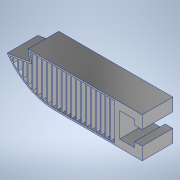
# Autodesk Inventor part: Finray_9_Kerbe_10deg
Saved by Autodesk Inventor 2022 (Build 260153000, 153)
## iProperties
Created: 2022-02-28
Part Number: Finray_9_Kerbe_10deg
Material: Generic
Document SubType Name: Modeling
Designer: richa
Density: 1 g/cm^3
Appearance: Aluminum - Flat
Author: richa
Autodesk Inventor part; units mm, degrees
ref_plane "YZ Plane" through (0, 0, 0) normal (1, 0, 0) x (0, 1, 0)
ref_plane "XZ Plane" through (0, 0, 0) normal (0, 1, 0) x (-1, 0, 0)
ref_plane "XY Plane" through (0, 0, 0) normal (0, 0, 1) x (1, 0, 0)
sketch "Sketch5" plane through (0, 0, 0) normal (0, 0, 1) x (1, 0, 0)
  line L0 (52.8, -15.6) -> (52.8, -10.6)
  line L1 (52.8, -10.6) -> (49.8, -10.6)
  line L2 (49.8, -10.6) -> (49.8, -12.6)
  line L3 (44, -12.6) -> (44, -3)
  line L4 (49.8, -3) -> (49.8, -5)
  line L5 (49.8, -5) -> (52.8, -5)
  line L6 (52.8, -5) -> (52.8, 0)
  line L7 (52.8, 0) -> (7.8, 0)
  line L8 (44, -3) -> (49.8, -3)
  line L9 (44, -12.6) -> (49.8, -12.6)
  line L10 (52.8, -15.6) -> (7.8, -15.6)
  line L11 (7.8, -15.6) -> (0, -15.6)
  line L12 (0, -15.6) -> (0, 0)
  line L13 (0, 0) -> (7.8, 0)
  point P0 (7.8, 0)
  dimension "d41" = 5.8
  dimension "d48" = 44
  dimension "d50" = 3
  dimension "d63" = 45
  dimension "d71" = 0
  dimension "d87" = 5.6
  dimension "d88" = 9.6
  dimension "d97" = 15.6
  constraints: 28 end point, 8 perpendicular, 4 collinear, 3 parallel, 2 horizontal, 1 vertical
  measures "d41" distance between parallel lines of L2 L3
  measures "d48" distance from line of L3 L12.end
  measures "d50" distance of L4.end L5.end
  measures "d63" distance of L0.start L10.end
  measures "d71" distance from line of L12.end L7
  measures "d87" distance from line of L0.end L5
  measures "d88" distance of L3.start L3.end
  measures "d97" distance of L11.end L12.end
extrude "Extrusion2" add sketch "Sketch5" along normal blind 12
sketch "Sketch8" plane through (0, 0, 0) normal (0, 0, -1) x (-1, 0, 0)
  line L0 (-8.1687, 0) -> (-8.8633, -3.9392)
  line L1 (-7.8, 0) -> (-1.143, 0) construction
  line L2 (0, -5.5021) -> (-8.8633, -3.9392)
  line L3 (-7.8, 0) -> (-8.1687, 0)
  line L4 (0, 0) -> (0, -15.6) projected
  line L5 (-52.8, 0) -> (0, 0) projected
  line L6 (-7.8, 0) -> (0, 0)
  line L7 (0, 0) -> (0, -5.5021)
  dimension "d80" = 100
  dimension "d95" = 4
  dimension "d96" = 9
  constraints: 12 end point, 2 collinear, 2 perpendicular, 1 horizontal, 1 point on line
  measures "d80" angle of L0 L1
  measures "d95" distance of L0.start L0.end
  measures "d96" distance of L2.start L0.end
extrude "Extrusion5" cut sketch "Sketch8" against normal through all
fillet "Fillet2" radius 23 1 edges at (0, -15.6, 6)
shell "Shell1" thickness 0.62 removed faces 1 at (23.9679, -7.5131, 12)
sketch "Sketch13" plane through (0, 0, 12) normal (0, 0, 1) x (1, 0, 0)
  line L0 (19.0404, -15.6) -> (52.8, -15.6) projected
  line L1 (42.0526, -15.6) -> (42.0526, 0)
  line L2 (52.8, 0) -> (8.1687, 0) projected
  line L3 (52.8, 0) -> (8.1687, 0) projected
  line L4 (52.8, -5) -> (52.8, 0) projected
  line L5 (49.8, -5) -> (52.8, -5) projected
  line L6 (49.8, -3) -> (49.8, -5) projected
  line L7 (44, -3) -> (49.8, -3) projected
  line L8 (44, -12.6) -> (44, -3) projected
  line L9 (49.8, -12.6) -> (44, -12.6) projected
  line L10 (49.8, -10.6) -> (49.8, -12.6) projected
  line L11 (52.8, -10.6) -> (49.8, -10.6) projected
  line L12 (52.8, -15.6) -> (52.8, -10.6) projected
  line L13 (42.0526, 0) -> (52.8, 0)
  line L14 (52.8, -5) -> (52.8, 0) projected
  line L15 (52.8, -5) -> (52.8, 0)
  line L16 (52.8, 0) -> (52.8, -5)
  line L17 (44, -12.6) -> (44, -3) projected
  line L18 (44, -3) -> (44, -12.6)
  line L19 (49.8, -12.6) -> (44, -12.6) projected
  line L20 (44, -12.6) -> (49.8, -12.6)
  line L21 (43.38, -13.22) -> (50.42, -13.22) projected
  line L22 (52.8, -10.6) -> (52.8, -15.6)
  line L23 (52.8, -15.6) -> (42.0526, -15.6)
  line L24 (44, -3) -> (49.8, -3) projected
  line L25 (44, -3) -> (49.8, -3)
  line L26 (49.8, -3) -> (49.8, -5)
  line L27 (49.8, -5) -> (52.8, -5)
  line L28 (52.8, -10.6) -> (49.8, -10.6)
  line L29 (49.8, -10.6) -> (49.8, -12.6)
  point P0 (0, 0)
  dimension "d102" = 10.7474
  constraints: 26 end point, 10 collinear, 2 point on line, 2 vertical, 1 parallel
  measures "d102" distance between parallel lines of L4 L1
extrude "Extrusion7" add sketch "Sketch13" against normal blind 12
sketch "Sketch14" plane through (8.9076, -0.62, 0.62) normal (0, 0, 1) x (1, 0, 0)
  line L0 (33.145, -14.36) -> (33.145, 0) projected
  line L1 (33.145, 0) -> (0, 0) projected
  line L2 (0.6739, -3.8221) -> (0, 0) projected
  line L3 (-7.835, -5.3225) -> (0.6739, -3.8221) projected
  arc A0 (-7.835, -5.3225) -> (10.1328, -14.36) centre (10.1328, 8.02) ccw projected
  line L4 (10.1328, -14.36) -> (33.145, -14.36) projected
  point P0 (-8.9076, 0.62)
extrude "Extrusion8" cut sketch "Sketch14" against normal blind 12
sketch "Sketch15" plane through (0, 0, 12) normal (0, 0, 1) x (1, 0, 0)
  line L0 (42.0526, -0.62) -> (8.9076, -0.62) construction
  line L1 (38.2426, -0.62) -> (38.6226, -0.62)
  line L2 (38.6226, -0.62) -> (38.6226, -14.98)
  line L3 (38.6226, -14.98) -> (38.2426, -14.98)
  line L4 (38.2426, -14.98) -> (38.2426, -0.62)
  line L5 (34.4326, -0.62) -> (34.8126, -0.62)
  line L6 (34.8126, -0.62) -> (34.8126, -14.98)
  line L7 (34.8126, -14.98) -> (34.4326, -14.98)
  line L8 (34.4326, -14.98) -> (34.4326, -0.62)
  line L9 (30.6226, -0.62) -> (31.0026, -0.62)
  line L10 (31.0026, -0.62) -> (31.0026, -14.98)
  line L11 (31.0026, -14.98) -> (30.6226, -14.98)
  line L12 (30.6226, -14.98) -> (30.6226, -0.62)
  line L13 (26.8126, -0.62) -> (27.1926, -0.62)
  line L14 (27.1926, -0.62) -> (27.1926, -14.98)
  line L15 (27.1926, -14.98) -> (26.8126, -14.98)
  line L16 (26.8126, -14.98) -> (26.8126, -0.62)
  line L17 (23.0026, -0.62) -> (23.3826, -0.62)
  line L18 (23.3826, -0.62) -> (23.3826, -14.98)
  line L19 (23.3826, -14.98) -> (23.0026, -14.98)
  line L20 (23.0026, -14.98) -> (23.0026, -0.62)
  line L21 (19.1926, -0.62) -> (19.5726, -0.62)
  line L22 (19.5726, -0.62) -> (19.5726, -14.98)
  line L23 (19.5726, -14.98) -> (19.1926, -14.98)
  line L24 (19.1926, -14.98) -> (19.1926, -0.62)
  line L25 (15.3826, -0.62) -> (15.7626, -0.62)
  line L26 (15.7626, -0.62) -> (15.7626, -14.98)
  line L27 (15.7626, -14.98) -> (15.3826, -14.98)
  line L28 (15.3826, -14.98) -> (15.3826, -0.62)
  line L29 (11.5726, -0.62) -> (11.9526, -0.62)
  line L30 (11.9526, -0.62) -> (11.9526, -14.4807)
  line L31 (11.5726, -14.3539) -> (11.5726, -0.62)
  arc A0 (1.0726, -5.9425) -> (19.0404, -14.98) centre (19.0404, 7.4) ccw projected
  line L32 (42.0526, -0.62) -> (42.0526, -14.98) projected
  line L33 (1.0726, -5.9425) -> (9.5815, -4.4421) construction
  arc A1 (0, -5.5021) -> (19.0404, -15.6) centre (19.0404, 7.4) ccw projected
  line L34 (8.1426, -4.6475) -> (7.7626, -4.6475)
  line L35 (7.7626, -4.6475) -> (7.7626, -12.5934)
  line L36 (7.7626, -12.5934) -> (8.1426, -12.5934)
  line L37 (8.1426, -12.5934) -> (8.1426, -4.6475)
  line L38 (42.0526, -14.98) -> (19.0404, -14.98) projected
  line L39 (40.1476, -14.98) -> (40.5276, -14.98)
  line L40 (40.5276, -14.98) -> (40.5276, -0.62)
  line L41 (40.5276, -0.62) -> (40.1476, -0.62)
  line L42 (40.1476, -0.62) -> (40.1476, -14.98)
  line L43 (36.3376, -0.62) -> (36.7176, -0.62)
  line L44 (36.7176, -0.62) -> (36.7176, -14.98)
  line L45 (36.7176, -14.98) -> (36.3376, -14.98)
  line L46 (36.3376, -14.98) -> (36.3376, -0.62)
  line L47 (32.5276, -0.62) -> (32.9076, -0.62)
  line L48 (32.9076, -0.62) -> (32.9076, -14.98)
  line L49 (32.9076, -14.98) -> (32.5276, -14.98)
  line L50 (32.5276, -14.98) -> (32.5276, -0.62)
  line L51 (28.7176, -0.62) -> (29.0976, -0.62)
  line L52 (29.0976, -0.62) -> (29.0976, -14.98)
  line L53 (29.0976, -14.98) -> (28.7176, -14.98)
  line L54 (28.7176, -14.98) -> (28.7176, -0.62)
  line L55 (24.9076, -0.62) -> (25.2876, -0.62)
  line L56 (25.2876, -0.62) -> (25.2876, -14.98)
  line L57 (25.2876, -14.98) -> (24.9076, -14.98)
  line L58 (24.9076, -14.98) -> (24.9076, -0.62)
  line L59 (21.0976, -0.62) -> (21.4776, -0.62)
  line L60 (21.4776, -0.62) -> (21.4776, -14.98)
  line L61 (21.4776, -14.98) -> (21.0976, -14.98)
  line L62 (21.0976, -14.98) -> (21.0976, -0.62)
  line L63 (17.2876, -0.62) -> (17.6676, -0.62)
  line L64 (17.6676, -0.62) -> (17.6676, -14.9379)
  line L65 (17.6676, -14.9379) -> (17.2876, -14.9379)
  line L66 (17.2876, -14.9379) -> (17.2876, -0.62)
  line L67 (13.4776, -0.62) -> (13.8576, -0.62)
  line L68 (13.8576, -0.62) -> (13.8576, -14.3716)
  line L69 (13.8576, -14.3716) -> (13.4776, -14.3716)
  line L70 (13.4776, -14.3716) -> (13.4776, -0.62)
  line L71 (9.6676, -0.62) -> (10.0476, -0.62)
  line L72 (10.0476, -0.62) -> (10.0476, -13.0938)
  line L73 (10.0476, -13.0938) -> (9.6676, -13.0938)
  line L74 (9.6676, -13.0938) -> (9.6676, -0.62)
  line L75 (2.4276, -5.7036) -> (2.0476, -5.7036)
  line L76 (2.0476, -5.7036) -> (2.0476, -7.799)
  line L77 (2.0476, -7.799) -> (2.4276, -7.799)
  line L78 (2.4276, -7.799) -> (2.4276, -5.7036)
  line L79 (6.2376, -5.0318) -> (5.8576, -5.0318)
  line L80 (5.8576, -5.0318) -> (5.8576, -11.3056)
  line L81 (6.2376, -11.3056) -> (6.2376, -5.0318)
  line L82 (39.8926, -14.98) -> (39.5126, -14.98)
  line L83 (36.0826, -14.98) -> (35.7026, -14.98)
  line L84 (32.2726, -14.98) -> (31.8926, -14.98)
  line L85 (28.4626, -14.98) -> (28.0826, -14.98)
  line L86 (24.6526, -14.98) -> (24.2726, -14.98)
  line L87 (5.8576, -11.3056) -> (6.2376, -11.3056)
  line L88 (4.3326, -9.9597) -> (3.9526, -9.9597)
  line L89 (3.9526, -9.9597) -> (3.9526, -5.1923)
  line L90 (3.9526, -5.1923) -> (4.3326, -5.1923)
  line L91 (4.3326, -5.1923) -> (4.3326, -9.9597)
  point P0 (0, 0)
  point P1 (11.5726, -13.6973)
  point P2 (11.9526, -13.828)
  dimension "d105" = 0.38
  dimension "d107" = 0.38
  dimension "d108" = 0.38
  dimension "d109" = 0.38
  dimension "d110" = 0.38
  dimension "d111" = 0.38
  dimension "d112" = 0.38
  dimension "d113" = 0.38
  dimension "d118" = 0.38
  dimension "d120" = 3.81
  dimension "d121" = 3.81
  dimension "d122" = 3.81
  dimension "d123" = 3.81
  dimension "d124" = 3.81
  dimension "d125" = 3.81
  dimension "d129" = 0.38
  dimension "d131" = 0.38
  dimension "d132" = 0.38
  dimension "d133" = 0.38
  dimension "d134" = 0.38
  dimension "d135" = 0.38
  dimension "d136" = 0.38
  dimension "d137" = 0.38
  dimension "d138" = 0.38
  dimension "d139" = 0.38
  dimension "d140" = 0.38
  dimension "d180" = 1.525
  dimension "d189" = 1.525
  dimension "d190" = 1.525
  dimension "d191" = 0.38
  dimension "d192" = 1.525
  dimension "d193" = 1.525
  dimension "d194" = 1.525
  dimension "d195" = 1.525
  dimension "d196" = 1.525
  dimension "d197" = 1.525
  dimension "d198" = 1.525
  dimension "d199" = 1.525
  dimension "d200" = 1.525
  dimension "d201" = 1.525
  dimension "d202" = 1.525
  dimension "d203" = 1.525
  constraints: 176 end point, 40 parallel, 22 perpendicular, 21 horizontal, 21 point on line, 5 point on circle, 7 other
  measures "d105" distance between parallel lines of L2 L4
  measures "d107" distance between parallel lines of L6 L8
  measures "d108" distance of L9.start L9.end
  measures "d109" distance of L13.start L13.end
  measures "d110" distance between parallel lines of L18 L20
  measures "d111" distance between parallel lines of L22 L24
  measures "d112" distance between parallel lines of L26 L28
  measures "d113" distance between parallel lines of L30 L31
  measures "d118" distance of L34.start L34.end
  measures "d120" distance between parallel lines of L12 L16
  measures "d121" distance between parallel lines of L16 L20
  measures "d122" distance between parallel lines of L20 L24
  measures "d123" distance between parallel lines of L24 L28
  measures "d124" distance between parallel lines of L28 L31
  measures "d125" distance between parallel lines of L31 L35
  measures "d129" distance between parallel lines of L40 L42
  measures "d131" distance between parallel lines of L44 L46
  measures "d132" distance between parallel lines of L48 L50
  measures "d133" distance between parallel lines of L52 L54
  measures "d134" distance between parallel lines of L56 L58
  measures "d135" distance between parallel lines of L60 L62
  measures "d136" distance between parallel lines of L64 L66
  measures "d137" distance between parallel lines of L68 L70
  measures "d138" distance between parallel lines of L72 L74
  measures "d139" distance between parallel lines of L81 L80
  measures "d140" distance between parallel lines of L78 L76
  measures "d180" distance between parallel lines of L35 L81
  measures "d189" distance between parallel lines of L40 L32
  measures "d190" distance between parallel lines of L2 L42
  measures "d191" distance between parallel lines of L91 L89
  measures "d192" distance between parallel lines of L44 L4
  measures "d193" distance between parallel lines of L46 L6
  measures "d194" distance between parallel lines of L8 L48
  measures "d195" distance between parallel lines of L50 L10
  measures "d196" distance between parallel lines of L52 L12
  measures "d197" distance between parallel lines of L56 L16
  measures "d198" distance between parallel lines of L60 L20
  measures "d199" distance between parallel lines of L64 L24
  measures "d200" distance between parallel lines of L28 L68
  measures "d201" distance between parallel lines of L31 L72
  measures "d202" distance between parallel lines of L80 L91
  measures "d203" distance between parallel lines of L89 L78
extrude "Extrusion9" add sketch "Sketch15" against normal blind 12 contours L1 L2 L3 L4 | L5 L6 L7 L8 | L9 L10 L11 L12 | L13 L14 L15 L16 | L17 L18 L19 L20 | L21 L22 L23 L24 | L25 L26 A0 L28 | A0 L26 L27 L28 | L29 L30 A0 L31 | L73 L74 A0 | A0 L74 L71 L72 | L89 A0 L91 L88 | L89 L90 L91 A0 | L37 L36 L35 A0 | A0 L35 L34 L37 | L80 L79 L81 A0 | A0 L81 L87 L80 | L76 L75 L78 A0 | A0 L78 L77 L76 | L70 L67 L68 A0 | A0 L69 L70 | L66 L63 L64 A0 | A0 L65 L66 | L38 L42 L41 L40 | L38 L46 L43 L44 | L38 L50 L47 L48 | L38 L54 L51 L52 | L38 L58 L55 L56 | L38 L62 L59 L60
equation "\"l1\" = 8"
equation "\"d1\" = 0.38"
body "Solid2"
